Autodesk Inventor part; units mm, degrees
(part 2 of 2)
  line L1383 (257, -13) -> (257, -22)
  line L1384 (258, -13) -> (267, -13)
  line L1385 (258, -22) -> (258, -13)
  line L1386 (267, -22) -> (258, -22)
  line L1387 (267, -13) -> (267, -22)
  line L1388 (268, -13) -> (277, -13)
  line L1389 (268, -22) -> (268, -13)
  line L1390 (277, -22) -> (268, -22)
  line L1391 (277, -13) -> (277, -22)
  line L1392 (278, -13) -> (287, -13)
  line L1393 (278, -22) -> (278, -13)
  line L1394 (287, -22) -> (278, -22)
  line L1395 (287, -13) -> (287, -22)
  line L1396 (288, -13) -> (297, -13)
  line L1397 (288, -22) -> (288, -13)
  line L1398 (297, -22) -> (288, -22)
  line L1399 (297, -13) -> (297, -22)
  line L1400 (298, -13) -> (307, -13)
  line L1401 (298, -22) -> (298, -13)
  line L1402 (307, -22) -> (298, -22)
  line L1403 (307, -13) -> (307, -22)
  line L1404 (308, -13) -> (317, -13)
  line L1405 (308, -22) -> (308, -13)
  line L1406 (317, -22) -> (308, -22)
  line L1407 (317, -13) -> (317, -22)
  line L1408 (-2, -23) -> (7, -23)
  line L1409 (-2, -32) -> (-2, -23)
  line L1410 (7, -32) -> (-2, -32)
  line L1411 (7, -23) -> (7, -32)
  line L1412 (8, -23) -> (17, -23)
  line L1413 (8, -32) -> (8, -23)
  line L1414 (17, -32) -> (8, -32)
  line L1415 (17, -23) -> (17, -32)
  line L1416 (18, -23) -> (27, -23)
  line L1417 (18, -32) -> (18, -23)
  line L1418 (27, -32) -> (18, -32)
  line L1419 (27, -23) -> (27, -32)
  line L1420 (28, -23) -> (37, -23)
  line L1421 (28, -32) -> (28, -23)
  line L1422 (37, -32) -> (28, -32)
  line L1423 (37, -23) -> (37, -32)
  line L1424 (38, -23) -> (47, -23)
  line L1425 (38, -32) -> (38, -23)
  line L1426 (47, -32) -> (38, -32)
  line L1427 (47, -23) -> (47, -32)
  line L1428 (48, -23) -> (57, -23)
  line L1429 (48, -32) -> (48, -23)
  line L1430 (57, -32) -> (48, -32)
  line L1431 (57, -23) -> (57, -32)
  line L1432 (58, -23) -> (67, -23)
  line L1433 (58, -32) -> (58, -23)
  line L1434 (67, -32) -> (58, -32)
  line L1435 (67, -23) -> (67, -32)
  line L1436 (68, -23) -> (77, -23)
  line L1437 (68, -32) -> (68, -23)
  line L1438 (77, -32) -> (68, -32)
  line L1439 (77, -23) -> (77, -32)
  line L1440 (78, -23) -> (87, -23)
  line L1441 (78, -32) -> (78, -23)
  line L1442 (87, -32) -> (78, -32)
  line L1443 (87, -23) -> (87, -32)
  line L1444 (88, -23) -> (97, -23)
  line L1445 (88, -32) -> (88, -23)
  line L1446 (97, -32) -> (88, -32)
  line L1447 (97, -23) -> (97, -32)
  line L1448 (98, -23) -> (107, -23)
  line L1449 (98, -32) -> (98, -23)
  line L1450 (107, -32) -> (98, -32)
  line L1451 (107, -23) -> (107, -32)
  line L1452 (108, -23) -> (117, -23)
  line L1453 (108, -32) -> (108, -23)
  line L1454 (117, -32) -> (108, -32)
  line L1455 (117, -23) -> (117, -32)
  line L1456 (118, -23) -> (127, -23)
  line L1457 (118, -32) -> (118, -23)
  line L1458 (127, -32) -> (118, -32)
  line L1459 (127, -23) -> (127, -32)
  line L1460 (128, -23) -> (137, -23)
  line L1461 (128, -32) -> (128, -23)
  line L1462 (137, -32) -> (128, -32)
  line L1463 (137, -23) -> (137, -32)
  line L1464 (138, -23) -> (147, -23)
  line L1465 (138, -32) -> (138, -23)
  line L1466 (147, -32) -> (138, -32)
  line L1467 (147, -23) -> (147, -32)
  line L1468 (148, -23) -> (157, -23)
  line L1469 (148, -32) -> (148, -23)
  line L1470 (157, -32) -> (148, -32)
  line L1471 (157, -23) -> (157, -32)
  line L1472 (158, -23) -> (167, -23)
  line L1473 (158, -32) -> (158, -23)
  line L1474 (167, -32) -> (158, -32)
  line L1475 (167, -23) -> (167, -32)
  line L1476 (168, -23) -> (177, -23)
  line L1477 (168, -32) -> (168, -23)
  line L1478 (177, -32) -> (168, -32)
  line L1479 (177, -23) -> (177, -32)
  line L1480 (178, -23) -> (187, -23)
  line L1481 (178, -32) -> (178, -23)
  line L1482 (187, -32) -> (178, -32)
  line L1483 (187, -23) -> (187, -32)
  line L1484 (188, -23) -> (197, -23)
  line L1485 (188, -32) -> (188, -23)
  line L1486 (197, -32) -> (188, -32)
  line L1487 (197, -23) -> (197, -32)
  line L1488 (198, -23) -> (207, -23)
  line L1489 (198, -32) -> (198, -23)
  line L1490 (207, -32) -> (198, -32)
  line L1491 (207, -23) -> (207, -32)
  line L1492 (208, -23) -> (217, -23)
  line L1493 (208, -32) -> (208, -23)
  line L1494 (217, -32) -> (208, -32)
  line L1495 (217, -23) -> (217, -32)
  line L1496 (218, -23) -> (227, -23)
  line L1497 (218, -32) -> (218, -23)
  line L1498 (227, -32) -> (218, -32)
  line L1499 (227, -23) -> (227, -32)
  line L1500 (228, -23) -> (237, -23)
  line L1501 (228, -32) -> (228, -23)
  line L1502 (237, -32) -> (228, -32)
  line L1503 (237, -23) -> (237, -32)
  line L1504 (238, -23) -> (247, -23)
  line L1505 (238, -32) -> (238, -23)
  line L1506 (247, -32) -> (238, -32)
  line L1507 (247, -23) -> (247, -32)
  line L1508 (248, -23) -> (257, -23)
  line L1509 (248, -32) -> (248, -23)
  line L1510 (257, -32) -> (248, -32)
  line L1511 (257, -23) -> (257, -32)
  line L1512 (258, -23) -> (267, -23)
  line L1513 (258, -32) -> (258, -23)
  line L1514 (267, -32) -> (258, -32)
  line L1515 (267, -23) -> (267, -32)
  line L1516 (268, -23) -> (277, -23)
  line L1517 (268, -32) -> (268, -23)
  line L1518 (277, -32) -> (268, -32)
  line L1519 (277, -23) -> (277, -32)
  line L1520 (278, -23) -> (287, -23)
  line L1521 (278, -32) -> (278, -23)
  line L1522 (287, -32) -> (278, -32)
  line L1523 (287, -23) -> (287, -32)
  line L1524 (288, -23) -> (297, -23)
  line L1525 (288, -32) -> (288, -23)
  line L1526 (297, -32) -> (288, -32)
  line L1527 (297, -23) -> (297, -32)
  line L1528 (298, -23) -> (307, -23)
  line L1529 (298, -32) -> (298, -23)
  line L1530 (307, -32) -> (298, -32)
  line L1531 (307, -23) -> (307, -32)
  line L1532 (308, -23) -> (317, -23)
  line L1533 (308, -32) -> (308, -23)
  line L1534 (317, -32) -> (308, -32)
  line L1535 (317, -23) -> (317, -32)
  line L1536 (-2, -33) -> (7, -33)
  line L1537 (-2, -42) -> (-2, -33)
  line L1538 (7, -42) -> (-2, -42)
  line L1539 (7, -33) -> (7, -42)
  line L1540 (8, -33) -> (17, -33)
  line L1541 (8, -42) -> (8, -33)
  line L1542 (17, -42) -> (8, -42)
  line L1543 (17, -33) -> (17, -42)
  line L1544 (18, -33) -> (27, -33)
  line L1545 (18, -42) -> (18, -33)
  line L1546 (27, -42) -> (18, -42)
  line L1547 (27, -33) -> (27, -42)
  line L1548 (28, -33) -> (37, -33)
  line L1549 (28, -42) -> (28, -33)
  line L1550 (37, -42) -> (28, -42)
  line L1551 (37, -33) -> (37, -42)
  line L1552 (38, -33) -> (47, -33)
  line L1553 (38, -42) -> (38, -33)
  line L1554 (47, -42) -> (38, -42)
  line L1555 (47, -33) -> (47, -42)
  line L1556 (48, -33) -> (57, -33)
  line L1557 (48, -42) -> (48, -33)
  line L1558 (57, -42) -> (48, -42)
  line L1559 (57, -33) -> (57, -42)
  line L1560 (58, -33) -> (67, -33)
  line L1561 (58, -42) -> (58, -33)
  line L1562 (67, -42) -> (58, -42)
  line L1563 (67, -33) -> (67, -42)
  line L1564 (68, -33) -> (77, -33)
  line L1565 (68, -42) -> (68, -33)
  line L1566 (77, -42) -> (68, -42)
  line L1567 (77, -33) -> (77, -42)
  line L1568 (78, -33) -> (87, -33)
  line L1569 (78, -42) -> (78, -33)
  line L1570 (87, -42) -> (78, -42)
  line L1571 (87, -33) -> (87, -42)
  line L1572 (88, -33) -> (97, -33)
  line L1573 (88, -42) -> (88, -33)
  line L1574 (97, -42) -> (88, -42)
  line L1575 (97, -33) -> (97, -42)
  line L1576 (98, -33) -> (107, -33)
  line L1577 (98, -42) -> (98, -33)
  line L1578 (107, -42) -> (98, -42)
  line L1579 (107, -33) -> (107, -42)
  line L1580 (108, -33) -> (117, -33)
  line L1581 (108, -42) -> (108, -33)
  line L1582 (117, -42) -> (108, -42)
  line L1583 (117, -33) -> (117, -42)
  line L1584 (118, -33) -> (127, -33)
  line L1585 (118, -42) -> (118, -33)
  line L1586 (127, -42) -> (118, -42)
  line L1587 (127, -33) -> (127, -42)
  line L1588 (128, -33) -> (137, -33)
  line L1589 (128, -42) -> (128, -33)
  line L1590 (137, -42) -> (128, -42)
  line L1591 (137, -33) -> (137, -42)
  line L1592 (138, -33) -> (147, -33)
  line L1593 (138, -42) -> (138, -33)
  line L1594 (147, -42) -> (138, -42)
  line L1595 (147, -33) -> (147, -42)
  line L1596 (148, -33) -> (157, -33)
  line L1597 (148, -42) -> (148, -33)
  line L1598 (157, -42) -> (148, -42)
  line L1599 (157, -33) -> (157, -42)
  line L1600 (158, -33) -> (167, -33)
  line L1601 (158, -42) -> (158, -33)
  line L1602 (167, -42) -> (158, -42)
  line L1603 (167, -33) -> (167, -42)
  line L1604 (168, -33) -> (177, -33)
  line L1605 (168, -42) -> (168, -33)
  line L1606 (177, -42) -> (168, -42)
  line L1607 (177, -33) -> (177, -42)
  line L1608 (178, -33) -> (187, -33)
  line L1609 (178, -42) -> (178, -33)
  line L1610 (187, -42) -> (178, -42)
  line L1611 (187, -33) -> (187, -42)
  line L1612 (188, -33) -> (197, -33)
  line L1613 (188, -42) -> (188, -33)
  line L1614 (197, -42) -> (188, -42)
  line L1615 (197, -33) -> (197, -42)
  line L1616 (198, -33) -> (207, -33)
  line L1617 (198, -42) -> (198, -33)
  line L1618 (207, -42) -> (198, -42)
  line L1619 (207, -33) -> (207, -42)
  line L1620 (208, -33) -> (217, -33)
  line L1621 (208, -42) -> (208, -33)
  line L1622 (217, -42) -> (208, -42)
  line L1623 (217, -33) -> (217, -42)
  line L1624 (218, -33) -> (227, -33)
  line L1625 (218, -42) -> (218, -33)
  line L1626 (227, -42) -> (218, -42)
  line L1627 (227, -33) -> (227, -42)
  line L1628 (228, -33) -> (237, -33)
  line L1629 (228, -42) -> (228, -33)
  line L1630 (237, -42) -> (228, -42)
  line L1631 (237, -33) -> (237, -42)
  line L1632 (238, -33) -> (247, -33)
  line L1633 (238, -42) -> (238, -33)
  line L1634 (247, -42) -> (238, -42)
  line L1635 (247, -33) -> (247, -42)
  line L1636 (248, -33) -> (257, -33)
  line L1637 (248, -42) -> (248, -33)
  line L1638 (257, -42) -> (248, -42)
  line L1639 (257, -33) -> (257, -42)
  line L1640 (258, -33) -> (267, -33)
  line L1641 (258, -42) -> (258, -33)
  line L1642 (267, -42) -> (258, -42)
  line L1643 (267, -33) -> (267, -42)
  line L1644 (268, -33) -> (277, -33)
  line L1645 (268, -42) -> (268, -33)
  line L1646 (277, -42) -> (268, -42)
  line L1647 (277, -33) -> (277, -42)
  line L1648 (278, -33) -> (287, -33)
  line L1649 (278, -42) -> (278, -33)
  line L1650 (287, -42) -> (278, -42)
  line L1651 (287, -33) -> (287, -42)
  line L1652 (288, -33) -> (297, -33)
  line L1653 (288, -42) -> (288, -33)
  line L1654 (297, -42) -> (288, -42)
  line L1655 (297, -33) -> (297, -42)
  line L1656 (298, -33) -> (307, -33)
  line L1657 (298, -42) -> (298, -33)
  line L1658 (307, -42) -> (298, -42)
  line L1659 (307, -33) -> (307, -42)
  line L1660 (308, -33) -> (317, -33)
  line L1661 (308, -42) -> (308, -33)
  line L1662 (317, -42) -> (308, -42)
  line L1663 (317, -33) -> (317, -42)
  line L1664 (-2, -43) -> (7, -43)
  line L1665 (-2, -52) -> (-2, -43)
  line L1666 (7, -52) -> (-2, -52)
  line L1667 (7, -43) -> (7, -52)
  line L1668 (8, -43) -> (17, -43)
  line L1669 (8, -52) -> (8, -43)
  line L1670 (17, -52) -> (8, -52)
  line L1671 (17, -43) -> (17, -52)
  line L1672 (18, -43) -> (27, -43)
  line L1673 (18, -52) -> (18, -43)
  line L1674 (27, -52) -> (18, -52)
  line L1675 (27, -43) -> (27, -52)
  line L1676 (28, -43) -> (37, -43)
  line L1677 (28, -52) -> (28, -43)
  line L1678 (37, -52) -> (28, -52)
  line L1679 (37, -43) -> (37, -52)
  line L1680 (38, -43) -> (47, -43)
  line L1681 (38, -52) -> (38, -43)
  line L1682 (47, -52) -> (38, -52)
  line L1683 (47, -43) -> (47, -52)
  line L1684 (48, -43) -> (57, -43)
  line L1685 (48, -52) -> (48, -43)
  line L1686 (57, -52) -> (48, -52)
  line L1687 (57, -43) -> (57, -52)
  line L1688 (58, -43) -> (67, -43)
  line L1689 (58, -52) -> (58, -43)
  line L1690 (67, -52) -> (58, -52)
  line L1691 (67, -43) -> (67, -52)
  line L1692 (68, -43) -> (77, -43)
  line L1693 (68, -52) -> (68, -43)
  line L1694 (77, -52) -> (68, -52)
  line L1695 (77, -43) -> (77, -52)
  line L1696 (78, -43) -> (87, -43)
  line L1697 (78, -52) -> (78, -43)
  line L1698 (87, -52) -> (78, -52)
  line L1699 (87, -43) -> (87, -52)
  line L1700 (88, -43) -> (97, -43)
  line L1701 (88, -52) -> (88, -43)
  line L1702 (97, -52) -> (88, -52)
  line L1703 (97, -43) -> (97, -52)
  line L1704 (98, -43) -> (107, -43)
  line L1705 (98, -52) -> (98, -43)
  line L1706 (107, -52) -> (98, -52)
  line L1707 (107, -43) -> (107, -52)
  line L1708 (108, -43) -> (117, -43)
  line L1709 (108, -52) -> (108, -43)
  line L1710 (117, -52) -> (108, -52)
  line L1711 (117, -43) -> (117, -52)
  line L1712 (118, -43) -> (127, -43)
  line L1713 (118, -52) -> (118, -43)
  line L1714 (127, -52) -> (118, -52)
  line L1715 (127, -43) -> (127, -52)
  line L1716 (128, -43) -> (137, -43)
  line L1717 (128, -52) -> (128, -43)
  line L1718 (137, -52) -> (128, -52)
  line L1719 (137, -43) -> (137, -52)
  line L1720 (138, -43) -> (147, -43)
  line L1721 (138, -52) -> (138, -43)
  line L1722 (147, -52) -> (138, -52)
  line L1723 (147, -43) -> (147, -52)
  line L1724 (148, -43) -> (157, -43)
  line L1725 (148, -52) -> (148, -43)
  line L1726 (157, -52) -> (148, -52)
  line L1727 (157, -43) -> (157, -52)
  line L1728 (158, -43) -> (167, -43)
  line L1729 (158, -52) -> (158, -43)
  line L1730 (167, -52) -> (158, -52)
  line L1731 (167, -43) -> (167, -52)
  line L1732 (168, -43) -> (177, -43)
  line L1733 (168, -52) -> (168, -43)
  line L1734 (177, -52) -> (168, -52)
  line L1735 (177, -43) -> (177, -52)
  line L1736 (178, -43) -> (187, -43)
  line L1737 (178, -52) -> (178, -43)
  line L1738 (187, -52) -> (178, -52)
  line L1739 (187, -43) -> (187, -52)
  line L1740 (188, -43) -> (197, -43)
  line L1741 (188, -52) -> (188, -43)
  line L1742 (197, -52) -> (188, -52)
  line L1743 (197, -43) -> (197, -52)
  line L1744 (198, -43) -> (207, -43)
  line L1745 (198, -52) -> (198, -43)
  line L1746 (207, -52) -> (198, -52)
  line L1747 (207, -43) -> (207, -52)
  line L1748 (208, -43) -> (217, -43)
  line L1749 (208, -52) -> (208, -43)
  line L1750 (217, -52) -> (208, -52)
  line L1751 (217, -43) -> (217, -52)
  line L1752 (218, -43) -> (227, -43)
  line L1753 (218, -52) -> (218, -43)
  line L1754 (227, -52) -> (218, -52)
  line L1755 (227, -43) -> (227, -52)
  line L1756 (228, -43) -> (237, -43)
  line L1757 (228, -52) -> (228, -43)
  line L1758 (237, -52) -> (228, -52)
  line L1759 (237, -43) -> (237, -52)
  line L1760 (238, -43) -> (247, -43)
  line L1761 (238, -52) -> (238, -43)
  line L1762 (247, -52) -> (238, -52)
  line L1763 (247, -43) -> (247, -52)
  line L1764 (248, -43) -> (257, -43)
  line L1765 (248, -52) -> (248, -43)
  line L1766 (257, -52) -> (248, -52)
  line L1767 (257, -43) -> (257, -52)
  line L1768 (258, -43) -> (267, -43)
  line L1769 (258, -52) -> (258, -43)
  line L1770 (267, -52) -> (258, -52)
  line L1771 (267, -43) -> (267, -52)
  line L1772 (268, -43) -> (277, -43)
  line L1773 (268, -52) -> (268, -43)
  line L1774 (277, -52) -> (268, -52)
  line L1775 (277, -43) -> (277, -52)
  line L1776 (278, -43) -> (287, -43)
  line L1777 (278, -52) -> (278, -43)
  line L1778 (287, -52) -> (278, -52)
  line L1779 (287, -43) -> (287, -52)
  line L1780 (288, -43) -> (297, -43)
  line L1781 (288, -52) -> (288, -43)
  line L1782 (297, -52) -> (288, -52)
  line L1783 (297, -43) -> (297, -52)
  line L1784 (298, -43) -> (307, -43)
  line L1785 (298, -52) -> (298, -43)
  line L1786 (307, -52) -> (298, -52)
  line L1787 (307, -43) -> (307, -52)
  line L1788 (308, -43) -> (317, -43)
  line L1789 (308, -52) -> (308, -43)
  line L1790 (317, -52) -> (308, -52)
  line L1791 (317, -43) -> (317, -52)
  line L1792 (-2, -53) -> (7, -53)
  line L1793 (-2, -62) -> (-2, -53)
  line L1794 (7, -62) -> (-2, -62)
  line L1795 (7, -53) -> (7, -62)
  line L1796 (8, -53) -> (17, -53)
  line L1797 (8, -62) -> (8, -53)
  line L1798 (17, -62) -> (8, -62)
  line L1799 (17, -53) -> (17, -62)
  line L1800 (18, -53) -> (27, -53)
  line L1801 (18, -62) -> (18, -53)
  line L1802 (27, -62) -> (18, -62)
  line L1803 (27, -53) -> (27, -62)
  line L1804 (28, -53) -> (37, -53)
  line L1805 (28, -62) -> (28, -53)
  line L1806 (37, -62) -> (28, -62)
  line L1807 (37, -53) -> (37, -62)
  line L1808 (38, -53) -> (47, -53)
  line L1809 (38, -62) -> (38, -53)
  line L1810 (47, -62) -> (38, -62)
  line L1811 (47, -53) -> (47, -62)
  line L1812 (48, -53) -> (57, -53)
  line L1813 (48, -62) -> (48, -53)
  line L1814 (57, -62) -> (48, -62)
  line L1815 (57, -53) -> (57, -62)
  line L1816 (58, -53) -> (67, -53)
  line L1817 (58, -62) -> (58, -53)
  line L1818 (67, -62) -> (58, -62)
  line L1819 (67, -53) -> (67, -62)
  line L1820 (68, -53) -> (77, -53)
  line L1821 (68, -62) -> (68, -53)
  line L1822 (77, -62) -> (68, -62)
  line L1823 (77, -53) -> (77, -62)
  line L1824 (78, -53) -> (87, -53)
  line L1825 (78, -62) -> (78, -53)
  line L1826 (87, -62) -> (78, -62)
  line L1827 (87, -53) -> (87, -62)
  line L1828 (88, -53) -> (97, -53)
  line L1829 (88, -62) -> (88, -53)
  line L1830 (97, -62) -> (88, -62)
  line L1831 (97, -53) -> (97, -62)
  line L1832 (98, -53) -> (107, -53)
  line L1833 (98, -62) -> (98, -53)
  line L1834 (107, -62) -> (98, -62)
  line L1835 (107, -53) -> (107, -62)
  line L1836 (108, -53) -> (117, -53)
  line L1837 (108, -62) -> (108, -53)
  line L1838 (117, -62) -> (108, -62)
  line L1839 (117, -53) -> (117, -62)
  line L1840 (118, -53) -> (127, -53)
  line L1841 (118, -62) -> (118, -53)
  line L1842 (127, -62) -> (118, -62)
  line L1843 (127, -53) -> (127, -62)
  line L1844 (128, -53) -> (137, -53)
  line L1845 (128, -62) -> (128, -53)
  line L1846 (137, -62) -> (128, -62)
  line L1847 (137, -53) -> (137, -62)
  line L1848 (138, -53) -> (147, -53)
  line L1849 (138, -62) -> (138, -53)
  line L1850 (147, -62) -> (138, -62)
  line L1851 (147, -53) -> (147, -62)
  line L1852 (148, -53) -> (157, -53)
  line L1853 (148, -62) -> (148, -53)
  line L1854 (157, -62) -> (148, -62)
  line L1855 (157, -53) -> (157, -62)
  line L1856 (158, -53) -> (167, -53)
  line L1857 (158, -62) -> (158, -53)
  line L1858 (167, -62) -> (158, -62)
  line L1859 (167, -53) -> (167, -62)
  line L1860 (168, -53) -> (177, -53)
  line L1861 (168, -62) -> (168, -53)
  line L1862 (177, -62) -> (168, -62)
  line L1863 (177, -53) -> (177, -62)
  line L1864 (178, -53) -> (187, -53)
  line L1865 (178, -62) -> (178, -53)
  line L1866 (187, -62) -> (178, -62)
  line L1867 (187, -53) -> (187, -62)
  line L1868 (188, -53) -> (197, -53)
  line L1869 (188, -62) -> (188, -53)
  line L1870 (197, -62) -> (188, -62)
  line L1871 (197, -53) -> (197, -62)
  line L1872 (198, -53) -> (207, -53)
  line L1873 (198, -62) -> (198, -53)
  line L1874 (207, -62) -> (198, -62)
  line L1875 (207, -53) -> (207, -62)
  line L1876 (208, -53) -> (217, -53)
  line L1877 (208, -62) -> (208, -53)
  line L1878 (217, -62) -> (208, -62)
  line L1879 (217, -53) -> (217, -62)
  line L1880 (218, -53) -> (227, -53)
  line L1881 (218, -62) -> (218, -53)
  line L1882 (227, -62) -> (218, -62)
  line L1883 (227, -53) -> (227, -62)
  line L1884 (228, -53) -> (237, -53)
  line L1885 (228, -62) -> (228, -53)
  line L1886 (237, -62) -> (228, -62)
  line L1887 (237, -53) -> (237, -62)
  line L1888 (238, -53) -> (247, -53)
  line L1889 (238, -62) -> (238, -53)
  line L1890 (247, -62) -> (238, -62)
  line L1891 (247, -53) -> (247, -62)
  line L1892 (248, -53) -> (257, -53)
  line L1893 (248, -62) -> (248, -53)
  line L1894 (257, -62) -> (248, -62)
  line L1895 (257, -53) -> (257, -62)
  line L1896 (258, -53) -> (267, -53)
  line L1897 (258, -62) -> (258, -53)
  line L1898 (267, -62) -> (258, -62)
  line L1899 (267, -53) -> (267, -62)
  line L1900 (268, -53) -> (277, -53)
  line L1901 (268, -62) -> (268, -53)
  line L1902 (277, -62) -> (268, -62)
  line L1903 (277, -53) -> (277, -62)
  line L1904 (278, -53) -> (287, -53)
  line L1905 (278, -62) -> (278, -53)
  line L1906 (287, -62) -> (278, -62)
  line L1907 (287, -53) -> (287, -62)
  line L1908 (288, -53) -> (297, -53)
  line L1909 (288, -62) -> (288, -53)
  line L1910 (297, -62) -> (288, -62)
  line L1911 (297, -53) -> (297, -62)
  line L1912 (298, -53) -> (307, -53)
  line L1913 (298, -62) -> (298, -53)
  line L1914 (307, -62) -> (298, -62)
  line L1915 (307, -53) -> (307, -62)
  line L1916 (308, -53) -> (317, -53)
  line L1917 (308, -62) -> (308, -53)
  line L1918 (317, -62) -> (308, -62)
  line L1919 (317, -53) -> (317, -62)
  line L1920 (-2, -63) -> (7, -63)
  line L1921 (-2, -72) -> (-2, -63)
  line L1922 (7, -72) -> (-2, -72)
  line L1923 (7, -63) -> (7, -72)
  line L1924 (8, -63) -> (17, -63)
  line L1925 (8, -72) -> (8, -63)
  line L1926 (17, -72) -> (8, -72)
  line L1927 (17, -63) -> (17, -72)
  line L1928 (18, -63) -> (27, -63)
  line L1929 (18, -72) -> (18, -63)
  line L1930 (27, -72) -> (18, -72)
  line L1931 (27, -63) -> (27, -72)
  line L1932 (28, -63) -> (37, -63)
  line L1933 (28, -72) -> (28, -63)
  line L1934 (37, -72) -> (28, -72)
  line L1935 (37, -63) -> (37, -72)
  line L1936 (38, -63) -> (47, -63)
  line L1937 (38, -72) -> (38, -63)
  line L1938 (47, -72) -> (38, -72)
  line L1939 (47, -63) -> (47, -72)
  line L1940 (48, -63) -> (57, -63)
  line L1941 (48, -72) -> (48, -63)
  line L1942 (57, -72) -> (48, -72)
  line L1943 (57, -63) -> (57, -72)
  line L1944 (58, -63) -> (67, -63)
  line L1945 (58, -72) -> (58, -63)
  line L1946 (67, -72) -> (58, -72)
  line L1947 (67, -63) -> (67, -72)
  line L1948 (68, -63) -> (77, -63)
  line L1949 (68, -72) -> (68, -63)
  line L1950 (77, -72) -> (68, -72)
  line L1951 (77, -63) -> (77, -72)
  line L1952 (78, -63) -> (87, -63)
  line L1953 (78, -72) -> (78, -63)
  line L1954 (87, -72) -> (78, -72)
  line L1955 (87, -63) -> (87, -72)
  line L1956 (88, -63) -> (97, -63)
  line L1957 (88, -72) -> (88, -63)
  line L1958 (97, -72) -> (88, -72)
  line L1959 (97, -63) -> (97, -72)
  line L1960 (98, -63) -> (107, -63)
  line L1961 (98, -72) -> (98, -63)
  line L1962 (107, -72) -> (98, -72)
  line L1963 (107, -63) -> (107, -72)
  line L1964 (108, -63) -> (117, -63)
  line L1965 (108, -72) -> (108, -63)
  line L1966 (117, -72) -> (108, -72)
  line L1967 (117, -63) -> (117, -72)
  line L1968 (118, -63) -> (127, -63)
  line L1969 (118, -72) -> (118, -63)
  line L1970 (127, -72) -> (118, -72)
  line L1971 (127, -63) -> (127, -72)
  line L1972 (128, -63) -> (137, -63)
  line L1973 (128, -72) -> (128, -63)
  line L1974 (137, -72) -> (128, -72)
  line L1975 (137, -63) -> (137, -72)
  line L1976 (138, -63) -> (147, -63)
  line L1977 (138, -72) -> (138, -63)
  line L1978 (147, -72) -> (138, -72)
  line L1979 (147, -63) -> (147, -72)
  line L1980 (148, -63) -> (157, -63)
  line L1981 (148, -72) -> (148, -63)
  line L1982 (157, -72) -> (148, -72)
  line L1983 (157, -63) -> (157, -72)
  line L1984 (158, -63) -> (167, -63)
  line L1985 (158, -72) -> (158, -63)
  line L1986 (167, -72) -> (158, -72)
  line L1987 (167, -63) -> (167, -72)
  line L1988 (168, -63) -> (177, -63)
  line L1989 (168, -72) -> (168, -63)
  line L1990 (177, -72) -> (168, -72)
  line L1991 (177, -63) -> (177, -72)
  line L1992 (178, -63) -> (187, -63)
  line L1993 (178, -72) -> (178, -63)
  line L1994 (187, -72) -> (178, -72)
  line L1995 (187, -63) -> (187, -72)
  line L1996 (188, -63) -> (197, -63)
  line L1997 (188, -72) -> (188, -63)
  line L1998 (197, -72) -> (188, -72)
  line L1999 (197, -63) -> (197, -72)
  line L2000 (198, -63) -> (207, -63)
  line L2001 (198, -72) -> (198, -63)
  line L2002 (207, -72) -> (198, -72)
  line L2003 (207, -63) -> (207, -72)
  line L2004 (208, -63) -> (217, -63)
  line L2005 (208, -72) -> (208, -63)
  line L2006 (217, -72) -> (208, -72)
  line L2007 (217, -63) -> (217, -72)
  line L2008 (218, -63) -> (227, -63)
  line L2009 (218, -72) -> (218, -63)
  line L2010 (227, -72) -> (218, -72)
  line L2011 (227, -63) -> (227, -72)
  line L2012 (228, -63) -> (237, -63)
  line L2013 (228, -72) -> (228, -63)
  line L2014 (237, -72) -> (228, -72)
  line L2015 (237, -63) -> (237, -72)
  line L2016 (238, -63) -> (247, -63)
  line L2017 (238, -72) -> (238, -63)
  line L2018 (247, -72) -> (238, -72)
  line L2019 (247, -63) -> (247, -72)
  line L2020 (248, -63) -> (257, -63)
  line L2021 (248, -72) -> (248, -63)
  line L2022 (257, -72) -> (248, -72)
  line L2023 (257, -63) -> (257, -72)
  line L2024 (258, -63) -> (267, -63)
  line L2025 (258, -72) -> (258, -63)
  line L2026 (267, -72) -> (258, -72)
  line L2027 (267, -63) -> (267, -72)
  line L2028 (268, -63) -> (277, -63)
  line L2029 (268, -72) -> (268, -63)
  line L2030 (277, -72) -> (268, -72)
  line L2031 (277, -63) -> (277, -72)
  line L2032 (278, -63) -> (287, -63)
  line L2033 (278, -72) -> (278, -63)
  line L2034 (287, -72) -> (278, -72)
  line L2035 (287, -63) -> (287, -72)
  line L2036 (288, -63) -> (297, -63)
  line L2037 (288, -72) -> (288, -63)
  line L2038 (297, -72) -> (288, -72)
  line L2039 (297, -63) -> (297, -72)
  line L2040 (298, -63) -> (307, -63)
  line L2041 (298, -72) -> (298, -63)
  line L2042 (307, -72) -> (298, -72)
  line L2043 (307, -63) -> (307, -72)
  line L2044 (308, -63) -> (317, -63)
  line L2045 (308, -72) -> (308, -63)
  line L2046 (317, -72) -> (308, -72)
  line L2047 (317, -63) -> (317, -72)
  line L2048 (-4, 9) -> (319, 9)
  line L2049 (319, 9) -> (319, -74)
  line L2050 (319, -74) -> (-4, -74)
  line L2051 (-4, -74) -> (-4, 9)
  dimension "d31" = 5
  dimension "d32" = 5
  dimension "d33" = 2
  dimension "d36" = 10
  dimension "d39" = 10
  dimension "d44" = 10
  dimension "d47" = 10
  dimension "d50" = 2
  dimension "d51" = 2
  dimension "d52" = 2
  dimension "d53" = 2
  constraints: 4104 end point, 6 parallel, 4 collinear, 4 horizontal, 3 perpendicular, 2 vertical, 4079 other
  measures "d31" distance of L2.end L1.end
  measures "d32" distance of L1.end L0.end
  measures "d33" distance between parallel lines of L2 L4
  measures "d36" distance of L1.end L9.end
  measures "d39" distance of L1.end L133.end
  measures "d44" distance of L4.start L1028.start
  measures "d47" distance of L4.start L1152.start
  measures "d50" distance between parallel lines of L1044 L2048
  measures "d51" distance between parallel lines of L1153 L2051
  measures "d52" distance between parallel lines of L2050 L1938
  measures "d53" distance between parallel lines of L2049 L1663
extrude "Extrusion3" add sketch "Sketch4" along normal blind 10 contours L2048 L2049 L2050 L2051
sketch "Sketch7" plane through (0, 0, 10) normal (0, 0, 1) x (1, 0, 0)
  circle A0 centre (-8, 13) radius 2.7
  line L0 (319, 9) -> (-4, 9) projected
  line L1 (-4, 9) -> (-4, -74) projected
  line L2 (-12, 17) -> (0, 17)
  line L3 (-12, 17) -> (-12, 5)
  line L4 (0, 17) -> (8, 9)
  line L5 (0, 17) -> (11.3137, 17) construction
  line L6 (-12, 5) -> (-4, -3)
  line L7 (-12, 5) -> (-0.6863, 5) construction
  line L8 (-4, -3) -> (-4, 9)
  line L9 (-4, 9) -> (8, 9)
  line L10 (157.5, -15.4696) -> (157.5, -28.6857)
  line L11 (109.5973, -32.5) -> (115.1342, -32.5)
  circle A1 centre (-8, -78) radius 2.7
  line L12 (-12, -82) -> (0, -82)
  line L13 (-12, -82) -> (-12, -70)
  line L14 (0, -82) -> (8, -74)
  line L15 (-12, -70) -> (-4, -62)
  line L16 (-4, -74) -> (8, -74)
  circle A2 centre (323, 13) radius 2.7
  line L17 (327, 17) -> (315, 17)
  line L18 (327, 17) -> (327, 5)
  line L19 (315, 17) -> (307, 9)
  line L20 (327, 5) -> (319, -3)
  line L21 (315, -82) -> (307, -74)
  line L22 (327, -82) -> (315, -82)
  line L23 (327, -82) -> (327, -70)
  line L24 (327, -70) -> (319, -62)
  circle A3 centre (323, -78) radius 2.7
  line L25 (319, -74) -> (319, 9) projected
  line L26 (307, 9) -> (319, 9)
  line L27 (319, 9) -> (319, -3)
  line L28 (319, -62) -> (319, -74)
  line L29 (-4, -74) -> (319, -74) projected
  line L30 (319, -74) -> (307, -74)
  line L31 (-4, -74) -> (-4, -62)
  line L32 (0, 17) -> (315, 17)
  line L33 (327, 5) -> (327, -70)
  line L34 (315, -82) -> (0, -82)
  line L35 (-12, -70) -> (-12, 5)
  point P0 (0, 0)
  point P1 (-4, -62)
  dimension "d64" = 5.4
  dimension "d65" = 4
  dimension "d66" = 4
  dimension "d67" = 8
  dimension "d68" = 8
  dimension "d71" = 45
  dimension "d72" = 45
  dimension "d73" = 161.5
  dimension "d74" = 41.5
  constraints: 64 end point, 18 symmetric about line, 5 horizontal, 4 centre point, 3 perpendicular, 3 vertical, 2 collinear, 2 equal length, 2 point on line, 3 other
  measures "d64" diameter of A0
  measures "d65" distance from line of L0 A0.centre
  measures "d66" distance from line of L1 A0.centre
  measures "d67" distance between parallel lines of L0 L2
  measures "d68" distance between parallel lines of L1 L3
  measures "d71" angle of L4 L5
  measures "d72" angle of L6 L7
  measures "d73" distance between parallel lines of L10 L1
  measures "d74" distance between parallel lines of L11 L0
extrude "Extrusion6" add sketch "Sketch7" against normal blind 2 contours L0 L19 L17 L18 L20 L25 | L0 L4 L32 L19 | L20 L33 L24 L25 | L0 L1 L6 L3 L2 L4 | L24 L23 L22 L21 L29 L25 | L1 L15 L35 L6 | L21 L34 L14 L29 | L1 L16 L14 L12 L13 L15
fillet "Fillet2" radius 3.8 4 edges at (327, 17, 9) (327, -82, 9) (-12, 17, 9) (-12, -82, 9)
body "Solid2"
